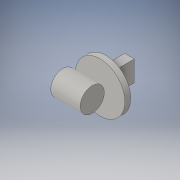
# Autodesk Inventor part: A2.5_Titus_RectangularPrisim
Saved by Autodesk Inventor 2016 (Build 200138000, 138)
## iProperties
Created: 2017-09-14
Part Number: A2.5_Titus_RectangularPrisim
Material: Generic
Document SubType Name: Modeling
Designer: sun01147
Density: 1 g/cm^3
Appearance: Default
Author: sun01147
Autodesk Inventor part; units mm, degrees
ref_plane "YZ Plane" through (0, 0, 0) normal (1, 0, 0) x (0, 1, 0)
ref_plane "XZ Plane" through (0, 0, 0) normal (0, 1, 0) x (-1, 0, 0)
ref_plane "XY Plane" through (0, 0, 0) normal (0, 0, 1) x (1, 0, 0)
sketch "Sketch1" plane through (0, 0, 0) normal (1, 0, 0) x (0, 1, 0)
  line L0 (16.0297, 0.2812) -> (15.9732, 0.2812)
  line L1 (15.9732, 0.2812) -> (15.9732, 0)
  line L2 (15.9732, 0) -> (16.0297, 0)
  line L3 (16.0297, 0) -> (16.0297, 0.2812)
  line L4 (94.7373, 0.2812) -> (0, 0.2812)
  line L5 (0, 0.2812) -> (0, -85.4009)
  line L6 (0, -85.4009) -> (94.7373, -85.4009)
  line L7 (94.7373, -85.4009) -> (94.7373, 0.2812)
  point P0 (0, 0)
  constraints: 16 end point, 4 parallel, 2 horizontal, 2 perpendicular
extrude "Extrusion1" add sketch "Sketch1" along normal blind 44.45 contours L4 L7 L6 L5 L1 L2 L3
sketch "Sketch2" plane through (44.45, 0, 0) normal (1, 0, 0) x (0, 0, -1)
  circle A0 centre (-242.3993, 165.5562) radius 55.2957
  point P0 (0, 0)
  constraints: 1 centre point
extrude "Extrusion2" add sketch "Sketch2" along normal blind 134.9375
sketch "Sketch3" plane through (0, 16.0297, 0.2812) normal (0, 0, 1) x (1, 0, 0)
  point P0 (0, -16.0297)
sketch "Sketch4" plane through (0, 16.0297, 0.2812) normal (0, 0, 1) x (1, 0, 0)
  circle A0 centre (0, 0) radius 113.7585
  point P0 (2.7076, 1.8404)
  constraints: 1 centre point
extrude "Extrusion3" add sketch "Sketch4" along normal blind 26.9875
body "Solid1"
